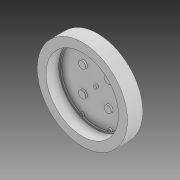
# Autodesk Inventor part: Shield
Saved by Autodesk Inventor 2020 (Build 240168000, 168)
## iProperties
Created: 2021-03-21
Part Number: Shield
Material: Generic
Document SubType Name: Modeling
Designer: DDeGo
Density: 1 g/cm^3
Appearance: Default
Author: DDeGo
Autodesk Inventor part; units mm, degrees
ref_plane "YZ Plane" through (0, 0, 0) normal (1, 0, 0) x (0, 1, 0)
ref_plane "XZ Plane" through (0, 0, 0) normal (0, 1, 0) x (-1, 0, 0)
ref_plane "XY Plane" through (0, 0, 0) normal (0, 0, 1) x (1, 0, 0)
sketch "Sketch1" plane through (0, 0, 0) normal (0, 0, 1) x (1, 0, 0)
  circle A0 centre (0, 0) radius 50
  line L0 (-19.5, -42.5) -> (19.5, -42.5) construction
  line L1 (19.5, -42.5) -> (19.5, 42.5) construction
  line L2 (19.5, 42.5) -> (-19.5, 42.5) construction
  line L3 (-19.5, 42.5) -> (-19.5, -42.5) construction
  line L4 (-19.5, -42.5) -> (19.5, 42.5) construction
  line L5 (19.5, -42.5) -> (-19.5, 42.5) construction
  circle A1 centre (-19.5, 42.5) radius 1.35
  circle A2 centre (19.5, 42.5) radius 1.35
  circle A3 centre (19.5, -42.5) radius 1.35
  circle A4 centre (-19.5, -42.5) radius 1.35
  dimension "d0" = 39
  dimension "d1" = 85
  dimension "d2" = 100
  dimension "d3" = 2.7
  constraints: 12 end point, 5 centre point, 5 coincident, 3 equal radius, 2 midpoint, 2 parallel, 1 horizontal, 1 perpendicular
  measures "d0" distance of L1.end L2.end
  measures "d1" distance of L0.end L1.end
  measures "d2" diameter of A0
  measures "d3" diameter of A4
extrude "Extrusion1" add sketch "Sketch1" along normal blind 1.5
sketch "Sketch2" plane through (0, 0, 1.5) normal (0, 0, 1) x (1, 0, 0)
  circle A0 centre (0, 0) radius 50 projected
  circle A1 centre (-19.5, 42.5) radius 1.35 projected
  arc A2 (-21.9946, 42.6642) -> (-17.9976, 44.4982) centre (-19.5, 42.5) ccw
  circle A3 centre (19.5, 42.5) radius 1.35 projected
  arc A4 (17.9976, 44.4982) -> (21.9946, 42.6642) centre (19.5, 42.5) ccw
  circle A5 centre (19.5, -42.5) radius 1.35 projected
  arc A6 (21.9946, -42.6642) -> (17.9976, -44.4982) centre (19.5, -42.5) ccw
  circle A7 centre (-19.5, -42.5) radius 1.35 projected
  arc A8 (-17.9976, -44.4982) -> (-21.9946, -42.6642) centre (-19.5, -42.5) ccw
  circle A9 centre (0, 0) radius 2.5
  circle A10 centre (-17.6777, 17.6777) radius 5
  line L0 (0, 0) -> (-17.6777, 17.6777) construction
  line L1 (0, 0) -> (-23.8881, 0) construction
  circle A11 centre (-17.6777, -17.6777) radius 5
  circle A12 centre (17.6777, -17.6777) radius 5
  circle A13 centre (17.6777, 17.6777) radius 5
  arc A14 (-17.9976, -44.4982) -> (17.9976, -44.4982) centre (0, 0) ccw
  arc A15 (-21.9946, 42.6642) -> (-21.9946, -42.6642) centre (0, 0) ccw
  arc A16 (21.9946, -42.6642) -> (21.9946, 42.6642) centre (0, 0) ccw
  arc A17 (17.9976, 44.4982) -> (-17.9976, 44.4982) centre (0, 0) ccw
  dimension "d6" = 5
  dimension "d8" = 5
  dimension "d9" = 10
  dimension "d10" = 25
  dimension "d11" = 45
  dimension "d14" = 360
  dimension "d16" = 2
  constraints: 16 point on circle, 13 centre point, 6 equal radius, 5 coincident, 4 end point, 1 horizontal, 9 other
  measures "d6" diameter of A2
  measures "d8" diameter of A9
  measures "d9" diameter of A10
  measures "d10" distance of L0.start L0.end
  measures "d11" angle of L0 L1
  measures "d16" radial gap between concentric circles of A0 A15
extrude "Extrusion2" add sketch "Sketch2" along normal blind 2.2
chamfer "Chamfer1" [suppressed]
sketch "Sketch3" plane through (0, 0, 0) normal (0, 0, -1) x (-1, 0, 0)
  circle A0 centre (0, 0) radius 2.5 construction
  line L0 (0, 0) -> (56.1, 0) construction
  circle A1 centre (56.1, 0) radius 5.1
  circle A2 centre (56.1, 0) radius 6.1 construction
  circle A3 centre (0, 0) radius 50 projected
  circle A4 centre (0, 0) radius 50 projected
  circle A5 centre (0, 0) radius 62.2
  circle A6 centre (45.3859, 32.9748) radius 5.1
  circle A7 centre (17.3359, 53.3543) radius 5.1
  circle A8 centre (-17.3359, 53.3543) radius 5.1
  circle A9 centre (-45.3859, 32.9748) radius 5.1
  circle A10 centre (-56.1, 0) radius 5.1
  circle A11 centre (-45.3859, -32.9748) radius 5.1
  circle A12 centre (-17.3359, -53.3543) radius 5.1
  circle A13 centre (17.3359, -53.3543) radius 5.1
  circle A14 centre (45.3859, -32.9748) radius 5.1
  point P0 (50, 0)
  dimension "d22" = 10.2
  dimension "d23" = 1
  dimension "d26" = 360
  constraints: 11 centre point, 3 coincident, 2 end point, 2 horizontal alignment, 1 horizontal, 1 point on line, 25 other
  measures "d22" diameter of A1
extrude "Extrusion3" add sketch "Sketch3" against normal blind 20.2
sketch "Sketch5" plane through (0, 0, 20.2) normal (0, 0, 1) x (1, 0, 0)
  circle A0 centre (0, 0) radius 62.2 projected
  circle A1 centre (0, 0) radius 50 projected
extrude "Extrusion5" add sketch "Sketch5" along normal blind 1
body "Solid1"
